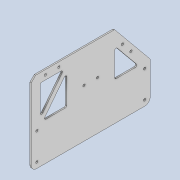
# Autodesk Inventor part: X Axis Belt V Wheel LEFT Outside Frame Machined No Logo
Saved by Autodesk Inventor 2022 (Build 260153000, 153)
## iProperties
Created: 2021-10-10
Part Number: X Axis Belt V Wheel LEFT Outside Frame Machined No Logo
Material: Generic
Document SubType Name: Modeling
Designer: Coy
Density: 1 g/cm^3
Appearance: Machined - Aluminum
Author: Coy
Autodesk Inventor part; units mm, degrees
ref_plane "YZ Plane" through (0, 0, 0) normal (1, 0, 0) x (0, 1, 0)
ref_plane "XZ Plane" through (0, 0, 0) normal (0, 1, 0) x (-1, 0, 0)
ref_plane "XY Plane" through (0, 0, 0) normal (0, 0, 1) x (1, 0, 0)
sketch "Sketch1" plane through (0, 0, 0) normal (1, 0, 0) x (0, 1, 0)
  line L0 (0, 0) -> (40, 0) construction
  line L1 (40, 0) -> (40, 66.5) construction
  line L2 (40, 66.5) -> (0, 66.5) construction
  line L3 (0, 66.5) -> (0, 0) construction
  line L4 (0, 66.5) -> (40, 66.5) construction
  line L5 (40, 66.5) -> (40, 86.5) construction
  line L6 (40, 86.5) -> (0, 86.5)
  line L7 (0, 86.5) -> (0, 66.5) construction
  line L8 (0, 0) -> (40, 0) construction
  line L9 (40, 0) -> (40, -20) construction
  line L10 (40, -20) -> (0, -20) construction
  line L11 (0, -20) -> (0, 0) construction
  line L12 (48.2, 61.45) -> (-8.2, 61.45) construction
  line L13 (-8.2, 61.45) -> (-8.2, 5.05) construction
  line L14 (-8.2, 5.05) -> (48.2, 5.05) construction
  line L15 (48.2, 5.05) -> (48.2, 61.45) construction
  line L16 (48.2, 33.25) -> (-8.2, 33.25) construction
  line L17 (40, 33.25) -> (0, 33.25) construction
  line L18 (43.57, 56.82) -> (-3.57, 56.82) construction
  line L19 (-3.57, 56.82) -> (-3.57, 9.68) construction
  line L20 (-3.57, 9.68) -> (43.57, 9.68) construction
  line L21 (43.57, 9.68) -> (43.57, 56.82) construction
  line L22 (43.57, 56.82) -> (48.2, 56.82) construction
  line L23 (43.57, 56.82) -> (43.57, 61.45) construction
  line L24 (-3.57, 9.68) -> (-8.2, 9.68) construction
  line L25 (-3.57, 9.68) -> (-3.57, 5.05) construction
  line L26 (40, -10) -> (0, -10) construction
  line L27 (40, 76.5) -> (0, 76.5) construction
  circle A0 centre (30, 76.5) radius 2.1
  circle A1 centre (10, 76.5) radius 2.1
  circle A2 centre (30, -10) radius 2.1
  circle A3 centre (10, -10) radius 2.1
  circle A4 centre (43.57, 56.82) radius 2.6
  circle A5 centre (43.57, 9.68) radius 2.6
  circle A6 centre (-3.57, 9.68) radius 2.6
  circle A7 centre (-3.57, 56.82) radius 2.6
  circle A8 centre (20, 33.25) radius 19.15
  circle A9 centre (-25, 18.25) radius 11.08 construction
  circle A10 centre (-25, 18.25) radius 13 construction
  circle A11 centre (-25, 18.25) radius 2.5
  line L28 (-60, 153.25) -> (-60, -86.75) construction
  circle A12 centre (-60, -86.75) radius 2.6
  circle A13 centre (-60, 153.25) radius 2.6
  line L29 (-120.2, 153.25) -> (-120.2, -86.75) construction
  circle A14 centre (-120.2, -86.75) radius 2.6
  circle A15 centre (-120.2, 153.25) radius 2.6
  circle A16 centre (-60, -86.75) radius 12 construction
  circle A17 centre (-120.2, -86.75) radius 12 construction
  circle A18 centre (-120.2, 153.25) radius 12 construction
  circle A19 centre (-60, 153.25) radius 12 construction
  line L30 (-110, 482.7599) -> (-70, 482.7599) construction
  line L31 (-70, -517.2401) -> (-110, -517.2401) construction
  circle A20 centre (-25, 48.25) radius 2.5
  circle A21 centre (-25, 48.25) radius 11.08 construction
  circle A22 centre (-25, 48.25) radius 13 construction
  circle A23 centre (20, 33.25) radius 11.08 construction
  circle A24 centre (20, 33.25) radius 13 construction
  line L32 (-23.1873, 29.1807) -> (18.1873, 22.3193) construction
  line L33 (18.1873, 44.1807) -> (-23.1873, 37.3193) construction
  line L34 (-120.8333, -99.25) -> (-47.8333, -99.25)
  line L35 (-47.8333, 165.75) -> (-120.8333, 165.75)
  line L36 (-132.8333, 153.75) -> (-132.8333, -87.25)
  line L37 (-60, 153.25) -> (-120.2, 153.25) construction
  line L38 (-120.2, -86.75) -> (-60, -86.75) construction
  line L39 (-60, 153.25) -> (-60, 165.75) construction
  line L40 (-120.2, -86.75) -> (-120.2, -99.25) construction
  line L41 (48.3276, -20) -> (48.3276, 86.5)
  line L42 (17.6122, 86.5) -> (40, 86.5) construction
  arc A25 (-120.8333, 165.75) -> (-132.8333, 153.75) centre (-120.8333, 153.75) ccw
  arc A26 (-132.8333, -87.25) -> (-120.8333, -99.25) centre (-120.8333, -87.25) ccw
  line L43 (48.3276, -20) -> (-47.8333, -99.25)
  line L44 (-47.8333, 165.75) -> (-47.8333, -99.25) construction
  line L45 (-120.2, -86.75) -> (-132.8333, -86.75) construction
  line L46 (-60, 153.25) -> (-47.8333, 153.25) construction
  line L47 (-36.08, 48.25) -> (-36.08, 286.613) construction
  line L48 (-47.8333, 145.75) -> (-47.8333, 86.5)
  line L49 (-47.8333, 86.5) -> (16.8804, 86.5)
  line L50 (-47.8333, -73.3332) -> (16.8804, -20)
  line L51 (-47.8333, -20) -> (16.8804, -20)
  line L52 (-47.8333, -73.3332) -> (-47.8333, -20)
  line L53 (48.3276, 86.5) -> (48.3276, 165.75)
  line L54 (48.3276, 165.75) -> (-47.8333, 165.75)
  line L55 (-47.8333, 145.75) -> (28.3276, 145.75)
  line L56 (28.3276, 145.75) -> (28.3276, 86.5)
  line L57 (-47.8333, 145.75) -> (28.3276, 86.5) construction
  line L58 (-39.6904, 145.75) -> (28.3276, 92.8349)
  line L59 (-47.8333, 139.4151) -> (20.1847, 86.5)
  point P0 (-132.8333, -99.25)
  point P1 (-132.8333, 165.75)
  point P2 (-47.8333, 139.8332)
  point P3 (0, 86.5)
  point P4 (0, 86.5)
  dimension "d190" = 22.16
  dimension "d165" = 40
  dimension "d166" = 66.5
  dimension "d167" = 40
  dimension "d168" = 20
  dimension "d169" = 40
  dimension "d170" = 20
  dimension "d171" = 56.4
  dimension "d172" = 56.4
  dimension "d173" = 0
  dimension "d174" = 8.2
  dimension "d175" = 47.14
  dimension "d176" = 47.14
  dimension "d177" = 4.2
  dimension "d178" = 20
  dimension "d179" = 10
  dimension "d180" = 10
  dimension "d181" = 20
  dimension "d182" = 4.2
  dimension "d183" = 4.2
  dimension "d184" = 4.2
  dimension "d185" = 5.2
  dimension "d186" = 5.2
  dimension "d187" = 5.2
  dimension "d188" = 5.2
  dimension "d189" = 38.3
  dimension "d191" = 26
  dimension "d192" = 5
  dimension "d193" = 240
  dimension "d194" = 60
  dimension "d195" = 5.2
  dimension "d196" = 5.2
  dimension "d197" = 5.2
  dimension "d198" = 5.2
  dimension "d199" = 60.2
  dimension "d200" = 24
  dimension "d201" = 24
  dimension "d202" = 24
  dimension "d203" = 24
  dimension "d204" = 40
  dimension "d205" = 1000
  dimension "d206" = 45
  dimension "d207" = 5
  dimension "d208" = 22.16
  dimension "d209" = 26
  dimension "d210" = 45
  dimension "d211" = 22.16
  dimension "d212" = 26
  dimension "d213" = 15
  dimension "d214" = 15
  dimension "d215" = 265
  dimension "d216" = 85
  dimension "d217" = 106.5
  dimension "d218" = 12
  dimension "d219" = 72.8333
  dimension "d220" = 28.3276
  dimension "d221" = 53.25
  dimension "d222" = 85
  dimension "d223" = 132.5
  dimension "d224" = 60.2
  dimension "d225" = 20
  dimension "d226" = 20
  dimension "d227" = 5
  dimension "d228" = 5
  constraints: 120 end point, 27 point on line, 26 centre point, 18 coincident, 18 parallel, 16 perpendicular, 9 horizontal, 9 midpoint, 8 point on circle, 8 tangent, 5 vertical, 3 symmetric about line, 1 equal radius, 4 other
  measures "d165" distance of L2.end L1.end
  measures "d166" distance of L1.end L0.end
  measures "d167" distance of L5.end L6.end
  measures "d168" distance of L5.end L4.end
  measures "d169" distance of L9.end L10.end
  measures "d170" distance of L9.end L8.end
  measures "d171" distance of L14.end L13.end
  measures "d172" distance of L13.end L12.end
  measures "d173" distance between parallel lines of L17 L16
  measures "d174" distance between parallel lines of L15 L1
  measures "d175" distance of L20.end L18.start
  measures "d176" distance of L19.end L20.end
  measures "d177" diameter of A0
  measures "d178" distance of A1.centre A0.centre
  measures "d179" distance from line of L5 A0.centre
  measures "d180" distance from line of L9 A2.centre
  measures "d181" distance of A2.centre A3.centre
  measures "d182" diameter of A1
  measures "d183" diameter of A2
  measures "d184" diameter of A3
  measures "d185" diameter of A4
  measures "d186" diameter of A5
  measures "d187" diameter of A6
  measures "d188" diameter of A7
  measures "d189" diameter of A8
  measures "d191" diameter of A10
  measures "d192" diameter of A11
  measures "d193" distance of L28.start L28.end
  measures "d194" distance between parallel lines of L7 L28
  measures "d195" diameter of A12
  measures "d196" diameter of A13
  measures "d197" diameter of A14
  measures "d198" diameter of A15
  measures "d199" distance between parallel lines of L28 L29
  measures "d200" diameter of A16
  measures "d201" diameter of A17
  measures "d202" diameter of A18
  measures "d203" diameter of A19
  measures "d204" distance of L31.start L31.end
  measures "d205" distance of L30.end L31.start
  measures "d206" horizontal distance of A8.centre point (-25, 18.25)
  measures "d207" diameter of A20
  measures "d208" diameter of A21
  measures "d209" diameter of A22
  measures "d210" horizontal distance of A8.centre A20.centre
  measures "d211" diameter of A23
  measures "d212" diameter of A24
  measures "d213" vertical distance of A8.centre A10.centre
  measures "d214" vertical distance of A23.centre A21.centre
  measures "d215" distance of point (-132.833, 165.75) point (-132.833, -99.25)
  measures "d216" distance of L35.start point (-132.833, 165.75)
  measures "d217" distance of L41.end L41.start
  measures "d218" radius of A25
  measures "d219" distance between parallel lines of L28 L36
  measures "d220" distance from line of A8.centre L41
  measures "d221" vertical distance of L41.end A23.centre
  measures "d222" distance of L34.end point (-132.833, -99.25)
  measures "d223" vertical distance of L35.start A24.centre
  measures "d224" distance of L37.start L37.end
  measures "d225" distance between parallel lines of L53 L56
  measures "d226" distance between parallel lines of L54 L55
  measures "d227" distance between parallel lines of L57 L58
  measures "d228" distance between parallel lines of L57 L59
extrude "Extrusion1" add sketch "Sketch1" along normal blind 3.175 contours L6 L59 L48 L55 L58 L56 | A0 | A1 | A2 | A3 | A4 | A5 | A6 | A7 | A8 | A26 L36 A25 L35 L54 L53 L41 L43 L34
sketch "Sketch6" plane through (3.175, 0, 0) normal (1, 0, 0) x (0, 0, -1)
  line L0 (20, 16.8804) -> (73.3332, -47.8333)
  line L1 (20, 16.8804) -> (73.3332, -47.8333)
  line L2 (39.0796, -6.2705) -> (54.5136, 6.4492) construction
  line L3 (99.25, -47.8333) -> (20, 48.3276)
  circle A0 centre (37.2568, 11.6648) radius 2.6
  circle A1 centre (56.3364, -11.4861) radius 2.6
  line L4 (37.2568, 11.6648) -> (46.7966, 0.0893) construction
  line L5 (56.3364, -11.4861) -> (46.7966, 0.0893) construction
  line L6 (-145.75, 28.3276) -> (-92.8349, 28.3276)
  line L7 (-119.2924, 28.3276) -> (-119.2924, 48.3276) construction
  line L8 (20, 48.3276) -> (-165.75, 48.3276) construction
  circle A2 centre (-104.2924, 38.3276) radius 2.6
  circle A3 centre (-134.2924, 38.3276) radius 2.6
  line L9 (-104.2924, 38.3276) -> (-119.2924, 38.3276) construction
  line L10 (-134.2924, 38.3276) -> (-119.2924, 38.3276) construction
  point P0 (0, 0)
  dimension "d229" = 5.2
  dimension "d230" = 5.2
  dimension "d231" = 15
  dimension "d232" = 15
  dimension "d233" = 30
  dimension "d234" = 5.2
  dimension "d235" = 5.2
  dimension "d236" = 15
  dimension "d237" = 15
  constraints: 22 end point, 5 perpendicular, 4 centre point, 3 midpoint, 3 point on line, 1 vertical
  measures "d229" diameter of A0
  measures "d230" diameter of A1
  measures "d231" distance of L4.start L4.end
  measures "d232" distance of L5.start L4.end
  measures "d233" distance from line of L0.start L2
  measures "d234" diameter of A2
  measures "d235" diameter of A3
  measures "d236" distance of L9.start L9.end
  measures "d237" distance of L10.start L9.end
extrude "Extrusion6" cut sketch "Sketch6" against normal through all
fillet "Fillet2" radius 3.175 11 edges at (1.5875, 28.3276, 92.8349) (1.5875, 20.1847, 86.5) (1.5875, 28.3276, 145.75) (1.5875, -39.6904, 145.75) (1.5875, -47.8333, 139.4151) (1.5875, -47.8333, 86.5) (1.5875, 48.3276, -20) (1.5875, 16.8804, -20) (1.5875, -47.8333, -20) (1.5875, -47.8333, -73.3332) (1.5875, -47.8333, -99.25)
chamfer "Chamfer1" distance 10 angle 45 1 edges at (1.5875, 48.3276, 165.75)
body "Solid1"
